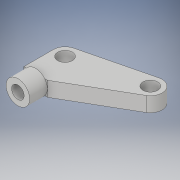
# Autodesk Inventor part: StteringArm
Saved by Autodesk Inventor 2018 (Build 220112000, 112)
## iProperties
Created: 2018-07-12
Part Number: StteringArm
Material: Generic
Document SubType Name: Modeling
Designer: Cole Tucker
Density: 1 g/cm^3
Appearance: Default
Author: Cole Tucker
Autodesk Inventor part; units mm, degrees
ref_plane "YZ Plane" through (0, 0, 0) normal (1, 0, 0) x (0, 1, 0)
ref_plane "XZ Plane" through (0, 0, 0) normal (0, 1, 0) x (-1, 0, 0)
ref_plane "XY Plane" through (0, 0, 0) normal (0, 0, 1) x (1, 0, 0)
sketch "Sketch1" plane through (0, 0, 0) normal (0, 1, 0) x (-1, 0, 0)
  circle A0 centre (0, 0) radius 3.175
  arc A1 (1.2165, -4.9322) -> (5.08, 0) centre (0, 0) ccw
  line L0 (5.08, 0) -> (5.08, 12.7)
  line L1 (0, 0) -> (-5.08, 0) construction
  line L2 (-5.08, 0) -> (-29.4214, -7.2565) construction
  line L3 (-5.08, 0) -> (20.32, 0) construction
  arc A2 (-31.9659, -2.8597) -> (-28.2049, -12.1887) centre (-29.4214, -7.2565) ccw
  circle A3 centre (-29.4214, -7.2565) radius 3.175
  line L4 (5.08, 12.7) -> (-5.08, 12.7)
  line L5 (-5.08, 12.7) -> (-31.9659, -2.8597)
  line L6 (1.2165, -4.9322) -> (-28.2049, -12.1887)
  dimension "d0" = 6.35
  dimension "d1" = 10.16
  dimension "d2" = 12.7
  dimension "d3" = 25.4
  dimension "d4" = 163.4
  dimension "d5" = 10.16
  dimension "d6" = 6.35
  dimension "d7" = 10.16
  constraints: 14 end point, 4 centre point, 4 coincident, 4 point on circle, 4 tangent, 3 horizontal, 1 equal length, 1 point on line, 1 vertical
  measures "d0" diameter of A0
  measures "d1" diameter of A1
  measures "d2" distance of L0.start L0.end
  measures "d3" distance of L1.end L2.end
  measures "d4" angle of L2 L3
  measures "d5" diameter of A2
  measures "d6" diameter of A3
  measures "d7" distance of L0.end L4.end
extrude "Extrusion1" add sketch "Sketch1" along normal blind 6.35
sketch "Sketch2" plane through (-5.08, 0, 12.7) normal (0, 0, 1) x (1, 0, 0)
  line L0 (5.08, 0) -> (5.08, 6.35) construction
  line L1 (0, 6.35) -> (10.16, 6.35) construction
  circle A0 centre (5.08, 3.175) radius 5.08
  dimension "d10" = 10.16
  constraints: 2 end point, 2 midpoint, 1 centre point
  measures "d10" diameter of A0
extrude "Extrusion2" add sketch "Sketch2" along normal blind 7.62
sketch "Sketch4" plane through (0, 3.175, 20.32) normal (0, 0, 1) x (1, 0, 0)
  point P0 (0, -3.175)
  point P1 (0, 0)
hole "Hole1" at (0, 3.175, 20.32) direction (0, 0, -1) diameter 5.3975 depth 10.16 tip angle 118
body "Solid1"
